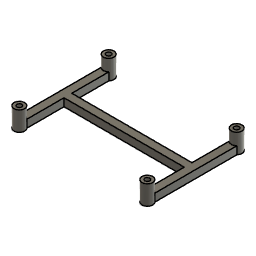
bracketCustomPcb (Autodesk Fusion 360 design; units mm, degrees)
Autodesk Fusion 360 part; units mm, degrees
sketch "Schizzo9" plane through (0, 0, 0) normal (0, 1, 0) x (1, 0, 0)
  line L0 (11, 28) -> (76.9, 28)
  line L1 (76.9, 28) -> (76.9, -18)
  line L2 (76.9, -18) -> (11, -18)
  line L3 (11, -18) -> (11, 28)
  circle A0 centre (11, 28) radius 2.75
  circle A1 centre (76.9, 28) radius 2.75
  circle A2 centre (11, -18) radius 2.75
  circle A3 centre (76.9, -18) radius 2.75
  line L4 (11, 28) -> (9, 28)
  line L5 (11, 28) -> (13, 28)
  line L6 (9, 28) -> (9, -18)
  line L7 (13, 28) -> (13, -18)
  line L8 (76.9, 28) -> (74.9, 28)
  line L9 (76.9, 28) -> (78.9, 28)
  line L10 (78.9, 28) -> (78.9, -18)
  line L11 (74.9, 28) -> (74.9, -18)
  line L12 (78.9, 5) -> (78.9, 7)
  line L13 (78.9, 5) -> (78.9, 3)
  line L14 (78.9, 7) -> (9, 7)
  line L15 (78.9, 3) -> (9, 3)
  dimension "d99" = 65.9
  dimension "d100" = 46
  dimension "d101" = 5.5
  dimension "d102" = 5.5
  dimension "d103" = 5.5
  dimension "d104" = 5.5
  dimension "d105" = 2
  dimension "d106" = 2
  dimension "d107" = 2
  dimension "d108" = 2
  dimension "d109" = 2
  dimension "d110" = 2
  constraint horizontal L0
  constraint vertical L1
  constraint horizontal L2
  constraint vertical L3
  constraint coincident L0.start L3.end
  constraint coincident L0.end L1.start
  constraint coincident L2.end L3.start
  constraint coincident L1.end L2.start
  constraint perpendicular L3 L4
  constraint perpendicular L3 L5
  constraint perpendicular L4 L6
  constraint coincident L2 L7.end
  constraint perpendicular L2 L7
  constraint perpendicular L1 L8
  constraint perpendicular L1 L9
  constraint perpendicular L9 L10
  constraint coincident L2 L11.end
  constraint perpendicular L2 L11
  constraint midpoint L10 L12.start
  constraint parallel L10 L12
  constraint parallel L10 L13
  constraint coincident L6 L14.end
  constraint perpendicular L6 L14
  constraint coincident L6 L15.end
  constraint perpendicular L6 L15
  measures "d99" distance of L0.start L0.end
  measures "d100" distance of L0.start L2.end
  measures "d101" diameter of A0
  measures "d102" diameter of A1
  measures "d103" diameter of A2
  measures "d104" diameter of A3
  measures "d105" distance of L0.start L4.end
  measures "d106" distance of L0.start L5.end
  measures "d107" distance of L0.end L8.end
  measures "d108" distance of L0.end L9.end
  measures "d109" distance of L12.start L12.end
  measures "d110" distance of L12.start L13.end
extrude "Estrusione16" add sketch "Schizzo9" along normal blind 4 contours L3 A0 L7 L14 | L3 A0 L6 L14 | L3 L7 L14 L15 | L3 L6 L14 L15 | L7 L11 L14 L15 | L3 A2 L7 L15 | L3 A2 L6 L15 | L1 A1 L11 L14 | L1 L11 L14 L15 | L1 A1 L10 L14 | L1 A3 L11 L15 | L1 L10 L12 L13 L14 L15 | L1 A3 L10 L15
extrude "Estrusione17" add sketch "Schizzo9" along normal blind 10 contours L0 A0 L4 L5 L6 | L0 L3 A0 L5 L7 | L3 A0 L4 L6 | L0 A0 L7 | L0 A1 L8 L9 L10 | L0 A1 L11 | L0 L1 A1 L8 L11 | L2 L3 A2 L7 | L2 L3 A2 | L1 A1 L9 L10 | L2 A2 L7 | L2 A3 L11 | L1 L2 A3 L11 | L1 L2 A3
hole "Foratura9" at (11, 10, -28) direction (0, -1, 0) diameter 2.5 depth 7 tip angle 118
hole "Foratura10" at (76.9, 10, -28) direction (0, -1, 0) diameter 2.5 depth 7 tip angle 118
hole "Foratura11" at (76.9, 10, 18) direction (0, -1, 0) diameter 2.5 depth 7 tip angle 118
hole "Foratura12" at (11, 10, 18) direction (0, -1, 0) diameter 2.5 depth 7 tip angle 118
